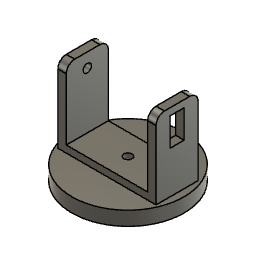
final assembly v2 (Autodesk Fusion 360 archive; units mm, degrees)
design "r1"
Autodesk Fusion 360 part; units mm, degrees
sketch "Sketch1" plane through (0, 0, 0) normal (0, 1, 0) x (1, 0, 0)
  circle A0 centre (0, 0) radius 40
  circle A1 centre (0, 0) radius 3
  dimension "d1" = 80
  dimension "d4" = 6
  constraint coincident A0.centre A1.centre
  constraint concentric A0 A1
  measures "d1" diameter of A0
  measures "d4" diameter of A1
extrude "Extrude2" add sketch "Sketch1" along normal blind 10
sketch "Sketch2" plane through (0, 10, 0) normal (0, 1, 0) x (-1, 0, 0)
  circle A0 centre (0, 0) radius 3
  circle A1 centre (0, 0) radius 40
  line L0 (-35, 15) -> (35, 15)
  line L1 (35, 15) -> (35, -15)
  line L2 (35, -15) -> (-35, -15)
  line L3 (-35, -15) -> (-35, 15)
  line L4 (-35, 15) -> (35, -15) construction
  line L5 (35, 15) -> (-35, -15) construction
  dimension "d7" = 70
  dimension "d8" = 30
  constraint horizontal L0
  constraint perpendicular L0 L1
  constraint parallel L0 L2
  constraint parallel L1 L3
  constraint coincident L4 A0.centre
  constraint coincident L5 A0.centre
  constraint coincident A0.centre A1.centre
  measures "d7" distance of L1.end L2.end
  measures "d8" distance of L0.end L1.end
extrude "Extrude3" add sketch "Sketch2" along normal blind 5 contours L0 L1 L2 L3
sketch "Sketch3" plane through (0, 15, 0) normal (0, 1, 0) x (-1, 0, 0)
  circle A0 centre (0, 0) radius 3
  line L0 (-35, -15) -> (35, -15)
  line L1 (35, -15) -> (35, 15)
  line L2 (35, 15) -> (-35, 15)
  line L3 (-35, 15) -> (-35, -15)
  line L4 (35, -15) -> (29, -15)
  line L5 (29, -15) -> (29, 15)
  line L6 (29, 15) -> (35, 15)
  line L7 (35, 15) -> (35, -15)
  line L8 (-35, -15) -> (-29, -15)
  line L9 (-29, -15) -> (-29, 15)
  line L10 (-29, 15) -> (-35, 15)
  line L11 (-35, 15) -> (-35, -15)
  dimension "d11" = 6
  dimension "d12" = 6
  dimension "d13" = 30
  dimension "d16" = 30
  constraint horizontal L4
  constraint vertical L5
  constraint horizontal L6
  constraint vertical L7
  constraint coincident L0.end L1.start
  constraint horizontal L8
  constraint vertical L9
  constraint horizontal L10
  constraint vertical L11
  constraint coincident L0.start L3.end
  measures "d7" distance of L2
  measures "d11" distance of L0.end L4.end L2
  measures "d12" distance of L0.start L8.end L2
  measures "d13" distance of L0.start L3.start L2
  measures "d16" distance of L4 L6
extrude "Extrude4" add sketch "Sketch3" along normal blind 50 contours L0 L2 L3 L8 L9 L10 L11 | L0 L1 L2 L4 L5 L6 L7
sketch "Sketch4" plane through (35, 0, 0) normal (1, 0, 0) x (0, 0, -1)
  line L0 (-15, 10) -> (15, 10)
  line L1 (15, 10) -> (15, 65)
  line L2 (15, 65) -> (-15, 65)
  line L3 (-15, 65) -> (-15, 10)
  line L4 (5, 40) -> (-5, 40)
  line L5 (-5, 40) -> (-5, 60)
  line L6 (-5, 60) -> (5, 60)
  line L7 (5, 60) -> (5, 40)
  line L8 (5, 40) -> (-5, 60) construction
  line L9 (-5, 40) -> (5, 60) construction
  point P0 (0, 50)
  dimension "d17" = 10
  dimension "d18" = 20
  constraint horizontal L4
  constraint perpendicular L4 L5
  constraint parallel L4 L6
  constraint parallel L5 L7
  constraint coincident L8 P0
  constraint coincident L9 P0
  measures "d17" distance of L5.end L6.end
  measures "d18" distance of L4.end L5.end
extrude "Extrude5" cut sketch "Sketch4" along normal up to surface (-6 mm away) and the other way blind 0 contours L4 L5 L6 L7
sketch "Sketch5" plane through (-35, 0, 0) normal (-1, 0, 0) x (0, 0, 1)
  line L0 (-15, 10) -> (15, 10)
  line L1 (15, 10) -> (15, 65)
  line L2 (15, 65) -> (-15, 65)
  line L3 (-15, 65) -> (-15, 10)
  circle A0 centre (0, 55) radius 3
  dimension "d23" = 6
  measures "d23" diameter of A0
extrude "Extrude6" cut sketch "Sketch5" against normal blind 20 contours A0
fillet "Fillet1" radius 6 4 edges at (32, 65, 15) (32, 65, -15) (-32, 65, 15) (-32, 65, -15)

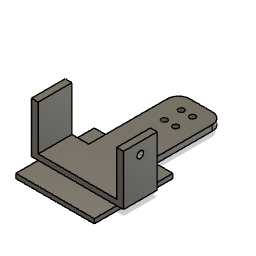
design "r2"
Autodesk Fusion 360 part; units mm, degrees
sketch "Sketch1" plane through (0, 0, 0) normal (0, 1, 0) x (1, 0, 0)
  line L0 (41, -15) -> (-41, -15)
  line L1 (-41, -15) -> (-41, 15)
  line L2 (-41, 15) -> (41, 15)
  line L3 (41, 15) -> (41, -15)
  line L4 (41, -15) -> (-41, 15) construction
  line L5 (-41, -15) -> (41, 15) construction
  dimension "d1" = 82
  dimension "d2" = 30
  constraint horizontal L0
  constraint perpendicular L0 L1
  constraint parallel L0 L2
  constraint parallel L1 L3
  constraint coincident L4 origin
  constraint coincident L5 origin
  measures "d1" distance of L1.end L2.end
  measures "d2" distance of L0.end L1.end
extrude "Extrude1" add sketch "Sketch1" along normal blind 5
sketch "Sketch2" plane through (0, 5, 0) normal (0, 1, 0) x (-1, 0, 0)
  line L0 (-41, -15) -> (41, -15)
  line L1 (41, -15) -> (41, 15)
  line L2 (41, 15) -> (-41, 15)
  line L3 (-41, 15) -> (-41, -15)
  line L4 (41, -15) -> (35, -15)
  line L5 (35, -15) -> (35, 15)
  line L6 (35, 15) -> (41, 15)
  line L7 (41, 15) -> (41, -15)
  line L8 (-41, -15) -> (-35, -15)
  line L9 (-35, -15) -> (-35, 15)
  line L10 (-35, 15) -> (-41, 15)
  line L11 (-41, 15) -> (-41, -15)
  constraint horizontal L4
  constraint vertical L5
  constraint horizontal L6
  constraint vertical L7
  constraint coincident L2 L5.end
  constraint coincident L0.end L1.start
  constraint horizontal L8
  constraint vertical L9
  constraint horizontal L10
  constraint vertical L11
  constraint coincident L0.start L3.end
extrude "Extrude2" add sketch "Sketch2" along normal blind 40 contours L0 L2 L3 L8 L9 L10 L11 | L0 L1 L2 L4 L5 L6 L7
sketch "Sketch3" plane through (41, 0, 0) normal (1, 0, 0) x (0, 0, -1)
  line L0 (-15, 0) -> (15, 0)
  line L1 (15, 0) -> (15, 45)
  line L2 (15, 45) -> (-15, 45)
  line L3 (-15, 45) -> (-15, 0)
  circle A0 centre (0, 35) radius 3
  dimension "d7" = 6
  dimension "d8" = 10
  measures "d7" diameter of A0
  measures "d8" distance of L2 A0.centre
extrude "Extrude3" cut sketch "Sketch3" against normal blind 10 contours A0
sketch "Sketch6" plane through (0, 0, 0) normal (0, 1, 0) x (1, 0, 0)
  line L0 (-10, 95) -> (10, 95)
  arc A0 (-10, 95) -> (-20, 85) centre (-10, 85) ccw
  line L1 (20, 15) -> (-20, 95) construction
  line L2 (-20, 15) -> (20, 95) construction
  arc A1 (20, 85) -> (10, 95) centre (10, 85) ccw
  line L3 (-20, 15) -> (-20, 85)
  line L4 (20, 85) -> (20, 15)
  line L5 (20, 15) -> (-20, 15)
  point P0 (0, 55)
  point P1 (0, 55)
  dimension "d19" = 40
  dimension "d20" = 80
  dimension "d21" = 10
  constraint horizontal L5
  constraint perpendicular L3 L5
  constraint parallel L0 L5
  constraint parallel L3 L4
  constraint coincident P1 L1
  constraint coincident P1 L2
  constraint coincident P1 P0
  constraint coincident L1.end L0
  constraint coincident L1.end L3
  constraint tangent L0 A0
  constraint tangent A0 L3
  constraint coincident L2.end L0
  constraint coincident L2.end L4
  constraint tangent L0 A1
  constraint tangent A1 L4
  constraint equal A0 A1
  measures "d19" distance of L2.end L1.end
  measures "d20" distance of L2.start L1.end
  measures "d21" radius of A0
extrude "Extrude6" add sketch "Sketch6" along normal blind 5
sketch "Sketch7" plane through (0, 0, 0) normal (0, -1, 0) x (1, 0, 0)
  line L0 (-41, -15) -> (-20, -15)
  line L1 (-20, -15) -> (-20, -85)
  arc A0 (-20, -85) -> (-10, -95) centre (-10, -85) ccw
  line L2 (-10, -95) -> (10, -95)
  arc A1 (10, -95) -> (20, -85) centre (10, -85) ccw
  line L3 (20, -85) -> (20, -15)
  line L4 (20, -15) -> (41, -15)
  line L5 (41, -15) -> (41, 15)
  line L6 (41, 15) -> (-41, 15)
  line L7 (-41, 15) -> (-41, -15)
  circle A2 centre (0, -75) radius 15
  dimension "d24" = 30
  measures "d24" diameter of A2
extrude "Extrude7" add sketch "Sketch7" along normal blind 5 contours A2
sketch "Sketch8" plane through (0, -5, 0) normal (0, -1, 0) x (1, 0, 0)
  circle A0 centre (0, -75) radius 15
  circle A1 centre (5.0873, -82.5589) radius 2.5
  circle A2 centre (-5.0873, -82.5589) radius 2.5
  circle A3 centre (5.0873, -67.4411) radius 2.5
  circle A4 centre (-5.0873, -67.4411) radius 2.5
  dimension "d27" = 5
  measures "d27" diameter of A1
extrude "Extrude8" cut sketch "Sketch8" against normal blind 17 contours A1 | A2 | A3 | A4
sketch "Sketch9" plane through (0, 0, 0) normal (0, -1, 0) x (1, 0, 0)
  circle A0 centre (0, -75) radius 15
  line L0 (-41, -15) -> (-20, -15)
  line L1 (-20, -15) -> (-20, -85)
  arc A1 (-20, -85) -> (-10, -95) centre (-10, -85) ccw
  line L2 (-10, -95) -> (10, -95)
  arc A2 (10, -95) -> (20, -85) centre (10, -85) ccw
  line L3 (20, -85) -> (20, -15)
  line L4 (20, -15) -> (41, -15)
  line L5 (41, -15) -> (41, 15)
  line L6 (41, 15) -> (-41, 15)
  line L7 (-41, 15) -> (-41, -15)
  line L8 (-35, 35) -> (35, 35)
  line L9 (35, 35) -> (35, -35)
  line L10 (35, -35) -> (-35, -35)
  line L11 (-35, -35) -> (-35, 35)
  line L12 (-35, 35) -> (35, -35) construction
  line L13 (35, 35) -> (-35, -35) construction
  dimension "d30" = 70
  dimension "d31" = 70
  constraint horizontal L8
  constraint perpendicular L8 L9
  constraint parallel L8 L10
  constraint parallel L9 L11
  constraint coincident L12 origin
  constraint coincident L13 origin
  measures "d30" distance of L9.end L10.end
  measures "d31" distance of L8.end L9.end
extrude "Extrude9" add sketch "Sketch9" along normal blind 4 contours L0 L1 L3 L4 L6 L9 L10 L11 | L0 L1 L10 L11 | L6 L8 L9 L11 | L3 L4 L9 L10

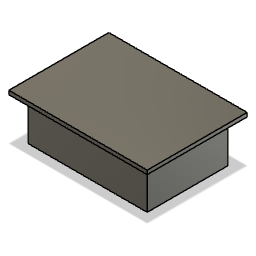
design "pcb cover"
Autodesk Fusion 360 part; units mm, degrees
sketch "Sketch1" plane through (0, 0, 0) normal (0, 1, 0) x (1, 0, 0)
  line L0 (77.5, -52.5) -> (-77.5, -52.5)
  line L1 (-77.5, -52.5) -> (-77.5, 52.5)
  line L2 (-77.5, 52.5) -> (77.5, 52.5)
  line L3 (77.5, 52.5) -> (77.5, -52.5)
  line L4 (77.5, -52.5) -> (-77.5, 52.5) construction
  line L5 (-77.5, -52.5) -> (77.5, 52.5) construction
  dimension "d1" = 155
  dimension "d2" = 105
  constraint horizontal L0
  constraint perpendicular L0 L1
  constraint parallel L0 L2
  constraint parallel L1 L3
  constraint coincident L4 origin
  constraint coincident L5 origin
  measures "d1" distance of L1.end L2.end
  measures "d2" distance of L0.end L1.end
extrude "Extrude1" add sketch "Sketch1" along normal blind 5
sketch "Sketch2" plane through (0, 5, 0) normal (0, 1, 0) x (-1, 0, 0)
  line L0 (-77.5, -52.5) -> (77.5, -52.5)
  line L1 (77.5, -52.5) -> (77.5, 52.5)
  line L2 (77.5, 52.5) -> (-77.5, 52.5)
  line L3 (-77.5, 52.5) -> (-77.5, -52.5)
  line L4 (-75, 50) -> (75, 50)
  line L5 (75, 50) -> (75, -50)
  line L6 (75, -50) -> (-75, -50)
  line L7 (-75, -50) -> (-75, 50)
  line L8 (-75, 50) -> (75, -50) construction
  line L9 (75, 50) -> (-75, -50) construction
  dimension "d5" = 150
  dimension "d6" = 100
  constraint horizontal L4
  constraint perpendicular L4 L5
  constraint parallel L4 L6
  constraint parallel L5 L7
  constraint coincident L8 origin
  constraint coincident L9 origin
  measures "d5" distance of L5.end L6.end
  measures "d6" distance of L4.end L5.end
extrude "Extrude2" add sketch "Sketch2" along normal blind 50
sketch "Sketch3" plane through (0, 0, 0) normal (0, -1, 0) x (1, 0, 0)
  line L0 (-77.5, -52.5) -> (77.5, -52.5)
  line L1 (77.5, -52.5) -> (77.5, 52.5)
  line L2 (77.5, 52.5) -> (-77.5, 52.5)
  line L3 (-77.5, 52.5) -> (-77.5, -52.5)
  circle A0 centre (0, 0) radius 3
  dimension "d9" = 6
  constraint coincident A0.centre origin
  measures "d9" diameter of A0
extrude "Extrude3" cut sketch "Sketch3" along normal through all and the other way through all contours A0
sketch "Sketch5" plane through (0, 55, 0) normal (0, 1, 0) x (-1, 0, 0)
  line L0 (75, -50) -> (-75, -50)
  line L1 (-75, -50) -> (-75, 50)
  line L2 (-75, 50) -> (75, 50)
  line L3 (75, 50) -> (75, -50)
  line L4 (-77.5, 52.5) -> (-77.5, -52.5)
  line L5 (-77.5, -52.5) -> (77.5, -52.5)
  line L6 (77.5, -52.5) -> (77.5, 52.5)
  line L7 (77.5, 52.5) -> (-77.5, 52.5)
  line L8 (90, 65) -> (-90, 65)
  line L9 (-90, 65) -> (-90, -65)
  line L10 (-90, -65) -> (90, -65)
  line L11 (90, -65) -> (90, 65)
  line L12 (90, 65) -> (-90, -65) construction
  line L13 (-90, 65) -> (90, -65) construction
  dimension "d24" = 180
  dimension "d25" = 130
  constraint horizontal L8
  constraint perpendicular L8 L9
  constraint parallel L8 L10
  constraint parallel L9 L11
  constraint coincident L12 origin
  constraint coincident L13 origin
  measures "d24" distance of L9.end L10.end
  measures "d25" distance of L8.end L9.end
extrude "Extrude5" add sketch "Sketch5" along normal blind 5 contours L0 L1 L2 L3 | L4 L5 L6 L7 | L8 L9 L10 L11
